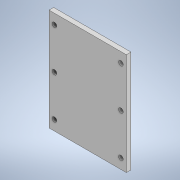
# Autodesk Inventor part: middle steel plate
Saved by Autodesk Inventor 2022 (Build 260153000, 153)
## iProperties
Created: 2023-03-21
Part Number: middle steel plate
Material: Generic
Document SubType Name: Modeling
Designer: chris
Density: 1 g/cm^3
Appearance: Default
Author: chris
Autodesk Inventor part; units mm, degrees
ref_plane "YZ Plane" through (0, 0, 0) normal (1, 0, 0) x (0, 1, 0)
ref_plane "XZ Plane" through (0, 0, 0) normal (0, 1, 0) x (-1, 0, 0)
ref_plane "XY Plane" through (0, 0, 0) normal (0, 0, 1) x (1, 0, 0)
sketch "Sketch1" plane through (0, 0, 0) normal (0, 0, 1) x (1, 0, 0)
  line L0 (0, 0) -> (0, 66)
  line L1 (0, 66) -> (36, 66)
  line L2 (36, 66) -> (36, 0)
  line L3 (36, 0) -> (0, 0)
  dimension "d0" = 66
  dimension "d1" = 36
  constraints: 8 end point, 2 perpendicular, 1 horizontal, 1 vertical
  measures "d0" distance of L0.start L0.end
  measures "d1" distance of L0.end L1.end
extrude "Extrusion1" add sketch "Sketch1" along normal blind 3
sketch "Sketch2" plane through (0, 0, 3) normal (0, 0, 1) x (1, 0, 0)
  line L0 (36, 66) -> (0, 66) projected
  line L1 (36, 66) -> (43, 66)
  line L2 (43, 66) -> (43, 0)
  line L3 (36, 0) -> (36, 66) projected
  line L4 (43, 0) -> (36, 0)
  line L5 (39.5, 66) -> (39.5, 59.5)
  line L6 (39.5, 0) -> (39.5, 6.5)
  line L7 (43, 33) -> (39.5, 33)
  circle A0 centre (39.5, 33) radius 1.5
  circle A1 centre (39.5, 59.5) radius 1.5
  circle A2 centre (39.5, 6.5) radius 1.5
  line L8 (18, 66) -> (18, 77.4734)
  line L9 (0, 66) -> (-7, 66)
  line L10 (-7, 66) -> (-7, 0)
  line L11 (-7, 0) -> (0, 0)
  line L12 (-3.5, 66) -> (-3.5, 59.5)
  line L13 (-3.5, 0) -> (-3.5, 6.5)
  line L14 (-7, 33) -> (-3.5, 33)
  circle A3 centre (-3.5, 33) radius 1.5
  circle A4 centre (-3.5, 59.5) radius 1.5
  circle A5 centre (-3.5, 6.5) radius 1.5
  line L15 (36, 0) -> (36, 66) projected
  line L16 (36, 66) -> (0, 66) projected
  line L17 (0, 66) -> (0, 0) projected
  line L18 (0, 0) -> (36, 0) projected
  dimension "d4" = 7
  dimension "d5" = 6.5
  dimension "d6" = 6.5
  dimension "d7" = 3
  dimension "d8" = 3
  dimension "d9" = 3
  constraints: 26 end point, 12 symmetric about line, 6 centre point, 6 coincident, 4 midpoint, 4 vertical, 2 horizontal, 1 perpendicular, 3 other
  measures "d4" distance of L0.start L1.end
  measures "d5" distance of L5.start L5.end
  measures "d6" distance of L6.start L6.end
  measures "d7" diameter of A0
  measures "d8" diameter of A1
  measures "d9" diameter of A2
extrude "Extrusion2" add sketch "Sketch2" against normal blind 3 contours L1 L2 L4 L3 | L17 L11 L10 L9
body "Solid1"
